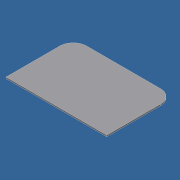
# Autodesk Inventor part: P1704_008_pcb
Saved by Autodesk Inventor 2019 (Build 230136000, 136)
## iProperties
Created: 2019-05-02
Part Number: P1704_008_pcb
Project: Nom Projet
Material: .
Description: Nom pièce
Document SubType Name: Modeling
Designer: Joan.MAILLARD
Authority: brut Ø
Density: 0.001 g/cm^3
Appearance: Par défaut
Material number: ---
Author: Joan.MAILLARD
Autodesk Inventor part; units mm, degrees
ref_plane "Plan YZ" through (0, 0, 0) normal (1, 0, 0) x (0, 1, 0)
ref_plane "Plan XZ" through (0, 0, 0) normal (0, 1, 0) x (-1, 0, 0)
ref_plane "Plan XY" through (0, 0, 0) normal (0, 0, 1) x (1, 0, 0)
sketch "Esquisse1" plane through (0, 0, 0) normal (0, 0, 1) x (1, 0, 0)
  line L0 (-75, -50) -> (75, -50)
  line L1 (-75, -50) -> (75, 50) construction
  line L2 (75, -50) -> (-75, 50) construction
  line L3 (-75, -50) -> (-75, 30)
  line L4 (75, 30) -> (75, -50)
  line L5 (75, 30) -> (75, 50) construction
  line L6 (55, 50) -> (75, 50) construction
  line L7 (-55, 50) -> (-75, 50) construction
  line L8 (-75, 30) -> (-75, 50) construction
  arc A0 (75, 30) -> (55, 50) centre (55, 30) ccw
  arc A1 (-55, 50) -> (-75, 30) centre (-55, 30) ccw
  line L9 (-55, 50) -> (55, 50)
  point P0 (0, 0)
  dimension "d0" = 150
  dimension "d1" = 100
  dimension "d23" = 20
  dimension "d24" = 20
  constraints: 20 end point, 4 point on circle, 4 tangent, 2 centre point, 2 collinear, 2 horizontal, 2 midpoint, 2 vertical, 1 perpendicular
  measures "d0" distance of L1.end L2.end
  measures "d1" distance of L0.end L1.end
  measures "d23" radius of A1
  measures "d24" radius of A0
extrude "Extrusion1" add sketch "Esquisse1" along normal blind 2
sketch "Esquisse7" plane through (0, 0, 0) normal (0, 0, -1) x (-1, 0, 0)
  line L0 (-62.5, 46.25) -> (-52.5, 46.25)
  line L1 (-52.5, 46.25) -> (-52.5, 11.25)
  line L2 (-52.5, 11.25) -> (-62.5, 11.25)
  line L3 (-62.5, 11.25) -> (-62.5, 46.25)
  line L4 (62.5, 46.25) -> (52.5, 46.25)
  line L5 (52.5, 46.25) -> (52.5, 11.25)
  line L6 (52.5, 11.25) -> (62.5, 11.25)
  line L7 (62.5, 11.25) -> (62.5, 46.25)
  line L8 (-75, -50) -> (-75, 30) projected
  line L9 (75, 30) -> (75, -50) projected
  line L10 (-55, 50) -> (55, 50) projected
  point P0 (0, 0)
  dimension "d4" = 10
  dimension "d6" = 10
  dimension "d7" = 35
  dimension "d8" = 35
  dimension "d20" = 12.5
  dimension "d21" = 12.5
  dimension "d22" = 3.75
  constraints: 16 end point, 4 parallel, 2 horizontal, 2 perpendicular, 1 point on line
  measures "d4" distance of L0.start L0.end
  measures "d6" distance of L4.start L4.end
  measures "d7" distance of L6.end L4.start
  measures "d8" distance between parallel lines of L2 L0
  measures "d20" distance between parallel lines of L8 L3
  measures "d21" distance between parallel lines of L9 L7
  measures "d22" distance between parallel lines of L10 L0
extrude "Extrusion2" add sketch "Esquisse7" along normal blind 6.5
equation "\"d6\" = d4"
equation "\"d7\" = d5"
equation "\"d21\" = d20"
equation "\"d5\" = 35"
